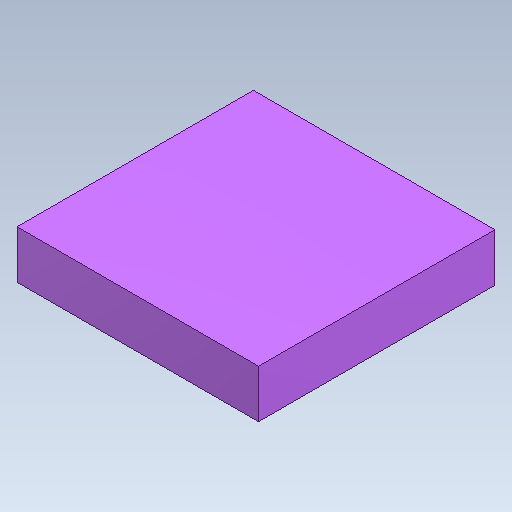
# Autodesk Inventor part: GREEN
Saved by Autodesk Inventor 2020 (Build 240168000, 168)
## iProperties
Created: 2019-05-24
Part Number: GREEN
Material: Generic
Document SubType Name: Modeling
Designer: psrob
Density: 1 g/cm^3
Appearance: 0603-LED-ALT1, GREEN
Author: psrob
Autodesk Inventor part; units mm, degrees
ref_plane "YZ Plane" through (0, 0, 0) normal (1, 0, 0) x (0, 1, 0)
ref_plane "XZ Plane" through (0, 0, 0) normal (0, 1, 0) x (-1, 0, 0)
ref_plane "XY Plane" through (0, 0, 0) normal (0, 0, 1) x (1, 0, 0)
sketch "0603-LED-ALT1, GREEN_20" plane through (0, 0, 0) normal (0, 0, 1) x (1, 0, 0)
  line L0 (-0.46, 0.2716) -> (0.5616, 0.2716)
  line L1 (0.5616, 0.2716) -> (0.5616, 0.0684)
  line L2 (0.5616, 0.0684) -> (-0.46, 0.0684)
  line L3 (-0.46, 0.0684) -> (-0.46, 0.2716)
  constraints: 8 end point
extrude "Extrusion1" add sketch "0603-LED-ALT1, GREEN_20" along normal blind 1
body "Solid1"
